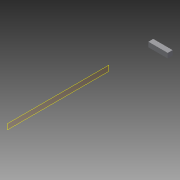
# Autodesk Inventor part: pillar
Saved by Autodesk Inventor 2015 (Build 190159000, 159)
## iProperties
Created: 2014-11-01
Part Number: pillar
Material: Generic
Document SubType Name: Modeling
Designer: jesse
Density: 1 g/cm^3
Appearance: Default
Author: jesse
Autodesk Inventor part; units mm, degrees
ref_plane "YZ Plane" through (0, 0, 0) normal (1, 0, 0) x (0, 1, 0)
ref_plane "XZ Plane" through (0, 0, 0) normal (0, 1, 0) x (-1, 0, 0)
ref_plane "XY Plane" through (0, 0, 0) normal (0, 0, 1) x (1, 0, 0)
ref_plane "Work Plane1" through (2543.3562, -205.1094, -195.9035) normal (1, 0, 0) x (0, 1, 0)
sketch "Sketch1" plane through (2543.3562, -205.1094, -195.9035) normal (1, 0, 0) x (0, 1, 0)
  line L0 (3.0798, -173.1143) -> (22.1298, -173.1143)
  line L1 (22.1298, -173.1143) -> (22.1298, -192.1643)
  line L2 (22.1298, -192.1643) -> (3.0798, -192.1643)
  line L3 (3.0798, -192.1643) -> (3.0798, -173.1143)
  point P0 (205.1094, 195.9035)
  dimension "d0" = 19.05
  dimension "d1" = 19.05
  constraints: 8 end point, 2 parallel, 1 horizontal, 1 perpendicular
  measures "d0" distance of L1.end L2.end
  measures "d1" distance of L0.end L1.end
extrude "Extrusion1" add sketch "Sketch1" along normal blind 76.2
body "Solid1"
